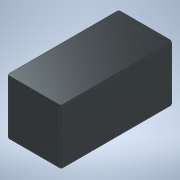
# Autodesk Inventor part: AC_power_box
Saved by Autodesk Inventor 2020 (Build 240168000, 168)
## iProperties
Created: 2022-08-31
Part Number: AC_power_box
Material: Iron, Cast
Document SubType Name: Modeling
Designer: Intuito_PC
Density: 7.15 g/cm^3
Appearance: Iron Gray
Author: Intuito_PC
Autodesk Inventor part; units mm, degrees
ref_plane "YZ Plane" through (0, 0, 0) normal (1, 0, 0) x (0, 1, 0)
ref_plane "XZ Plane" through (0, 0, 0) normal (0, 1, 0) x (-1, 0, 0)
ref_plane "XY Plane" through (0, 0, 0) normal (0, 0, 1) x (1, 0, 0)
sketch "Sketch1" plane through (0, 0, 0) normal (0, 0, 1) x (1, 0, 0)
  line L0 (0, 0) -> (-85, 0)
  line L1 (-85, 0) -> (-85, 85)
  line L2 (-85, 85) -> (0, 85)
  line L3 (0, 85) -> (0, 0)
  dimension "d0" = 85
  dimension "d1" = 85
  constraints: 8 end point, 2 parallel, 1 horizontal, 1 perpendicular
  measures "d0" distance of L1.end L2.end
  measures "d1" distance of L0.end L1.end
extrude "Extrusion1" add sketch "Sketch1" along normal blind 175
fillet "Fillet2" radius 3.175 8 edges at (-85, 42.5, 175) (0, 42.5, 175) (-42.5, 0, 175) (-85, 0, 87.5) (0, 0, 87.5) (0, 42.5, 0) (-42.5, 0, 0) (-85, 42.5, 0)
shell "Shell1" thickness 2.54 removed faces 1 at (-28.3333, 85, 59.3917)
sketch "Sketch2" plane through (-81.825, 85, 0) normal (0, 1, 0) x (1, 0, 0)
  line L0 (-2.54, -175) -> (81.19, -175)
  line L1 (81.19, -175) -> (81.19, -0.635)
  line L2 (81.19, -0.635) -> (-2.54, -0.635)
  line L3 (-2.54, -0.635) -> (-2.54, -175)
  point P0 (81.825, 0)
  point P1 (0, -172.46)
  point P2 (78.65, -3.175)
  constraints: 8 end point, 2 parallel, 1 perpendicular
extrude "Extrusion2" add sketch "Sketch2" along normal blind 2.54
fillet "Fillet3" radius 3.175 4 edges at (-84.365, 86.27, 175) (-0.635, 86.27, 175) (-0.635, 86.27, 0.635) (-84.365, 86.27, 0.635)
body "Solid1"
